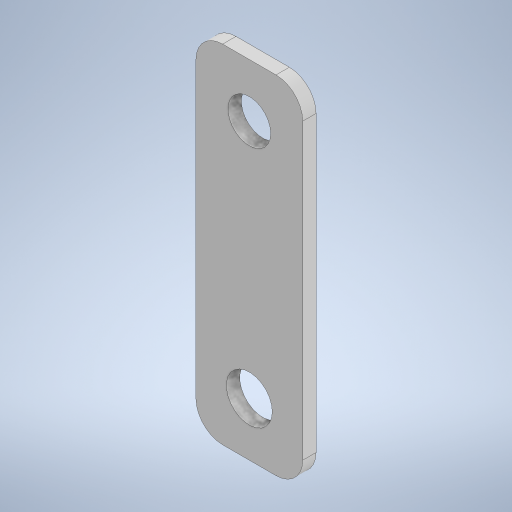
# Autodesk Inventor part: Servo horn
Saved by Autodesk Inventor 2023 (Build 270158000, 158)
## iProperties
Created: 2022-07-18
Part Number: Servo horn
Material: Generic
Document SubType Name: Sheet Metal
Designer: earls
Density: 1 g/cm^3
Sheet Metal Rule: Default_mm
Appearance: Default
Author: earls
Autodesk Inventor part; units mm, degrees
ref_plane "YZ Plane" through (0, 0, 0) normal (1, 0, 0) x (0, 1, 0)
ref_plane "XZ Plane" through (0, 0, 0) normal (0, 1, 0) x (-1, 0, 0)
ref_plane "XY Plane" through (0, 0, 0) normal (0, 0, 1) x (1, 0, 0)
sketch "Sketch1" plane through (0, 0, 0) normal (0, 0, 1) x (1, 0, 0)
  line L0 (-5, 65) -> (-15, 65)
  arc A0 (-15, 65) -> (-20, 60) centre (-15, 60) ccw
  line L1 (-20, 60) -> (-20, 5)
  arc A1 (-20, 5) -> (-15, 0) centre (-15, 5) ccw
  line L2 (-15, 0) -> (-5, 0)
  arc A2 (-5, 0) -> (0, 5) centre (-5, 5) ccw
  line L3 (0, 5) -> (0, 60)
  arc A3 (0, 60) -> (-5, 65) centre (-5, 60) ccw
  circle A4 centre (-10, 10) radius 4.3
  circle A5 centre (-10, 55) radius 4
  point P0 (0, 0)
  point P1 (0, 0)
  dimension "d0" = 8
  dimension "d1" = 8.6
  measures "d0" diameter of A5
  measures "d1" diameter of A4
extrude "Plate1" add sketch "Sketch1" along normal blind 2.5
equation "\"d2\" = Thickness"
equation "\"BendRadius\" = Thickness"
equation "\"BendReliefWidth\" = Thickness"
equation "\"BendReliefDepth\" = 0.5 * Thickness"
equation "\"MinimumRemnant\" = 2 * Thickness"
equation "\"TransitionRadius\" = BendRadius"
equation "\"JacobiRadiusSize\" = BendRadius"
equation "\"GapSize\" = Thickness"
equation "\"Thickness\" = 2.5"
body "Solid1"
